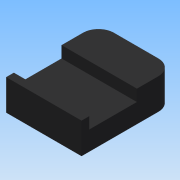
# Autodesk Inventor part: натяжитель ремня
Saved by Autodesk Inventor 2017 (Build 210142000, 142)
## iProperties
Part Number: натяжитель ремня
Material: Типовые
Document SubType Name: Modeling
Designer: Max
Mass: 0.473949 g
Surface Area: 4.70876 cm^2
Volume: 0.473949 cm^3
Density: 1 g/cm^3
Appearance: Резина — черная
Author: Max
Autodesk Inventor part; units mm, degrees
ref_plane "YZ Plane" through (0, 0, 0) normal (1, 0, 0) x (0, 1, 0)
ref_plane "XZ Plane" through (0, 0, 0) normal (0, 1, 0) x (-1, 0, 0)
ref_plane "XY Plane" through (0, 0, 0) normal (0, 0, 1) x (1, 0, 0)
sketch "Эскиз1" plane through (0, 0, 0) normal (0, 0, 1) x (1, 0, 0)
  arc A0 (9.8, 10) -> (7.8, 12) centre (7.8, 10) ccw projected
  line L0 (2, 12) -> (7.8, 12) projected
  arc A1 (2, 12) -> (0, 10) centre (2, 10) ccw projected
  line L1 (0, 0) -> (0, 10) projected
  line L2 (9.8, 0) -> (0, 0) projected
  line L3 (9.8, 0) -> (9.8, 10) projected
  line L4 (2.05, 7.1454) -> (4.9, 8.7909) projected
  line L5 (4.9, 8.7909) -> (7.75, 7.1454) projected
  line L6 (7.75, 7.1454) -> (7.75, 3.8546) projected
  line L7 (7.75, 3.8546) -> (4.9, 2.2091) projected
  line L8 (4.9, 2.2091) -> (2.05, 3.8546) projected
  line L9 (2.05, 3.8546) -> (2.05, 7.1454) projected
  circle A2 centre (4.9, 5.5) radius 1.7 projected
  circle A3 centre (4.9, 5.5) radius 1.5
  dimension "d0" = 3
  constraints: 1 centre point, 1 coincident
  measures "d0" diameter of A3
extrude "Выдавливание1" add sketch "Эскиз1" along normal blind 4.2 contours L3 L2 L1 A1 L0 A0 | L4 L5 L6 L7 L8 L9 | A2 | A3
sketch "Эскиз2" plane through (0, 0, 4.2) normal (0, 0, 1) x (1, 0, 0)
  line L0 (0, 10) -> (0, 0) projected
  line L1 (9.8, 0) -> (9.8, 10) projected
  line L2 (0, 7.2) -> (9.8, 7.2)
  line L3 (9.8, 7.2) -> (9.8, 1)
  line L4 (9.8, 1) -> (0, 1)
  line L5 (0, 1) -> (0, 7.2)
  line L6 (0, 0) -> (9.8, 0) projected
  dimension "d3" = 1
  dimension "d4" = 6.2
  constraints: 8 end point, 2 parallel, 2 point on line, 1 horizontal, 1 perpendicular
  measures "d3" distance between parallel lines of L6 L4
  measures "d4" distance between parallel lines of L4 L2
extrude "Выдавливание2" cut sketch "Эскиз2" against normal blind 1 contours L2 L1 L4 L0
sketch "Эскиз3" plane through (2, 12, 0) normal (0, 1, 0) x (1, 0, 0)
  line L0 (5.8, 0) -> (5.8, -4.2) projected
  line L1 (0, 0) -> (5.8, 0) projected
  line L2 (5.8, 0) -> (0, 0)
  line L3 (2.9, 0) -> (2.9, -1.6661)
  line L4 (3.9, 0) -> (1.9, 0)
  line L5 (1.9, 0) -> (1.9, -1)
  line L6 (1.9, -1) -> (3.9, -1)
  line L7 (3.9, -1) -> (3.9, 0)
  line L8 (3.9, 0) -> (1.9, 0)
  line L9 (1.9, 0) -> (1.9, 2)
  line L10 (1.9, 2) -> (3.9, 2)
  line L11 (3.9, 2) -> (3.9, 0)
  point P0 (-2, 0)
  dimension "d7" = 2
  dimension "d8" = 1
  dimension "d9" = 2
  constraints: 20 end point, 5 equal length, 2 horizontal, 2 perpendicular, 1 midpoint, 1 point on line, 1 vertical, 1 other
  measures "d7" distance between parallel lines of L5 L7
  measures "d8" distance between parallel lines of L1 L6
  measures "d9" distance from line of L3.start L10
extrude "Выдавливание3" add sketch "Эскиз3" against normal up to surface (12 mm away) contours L9 L10 L11 L1
